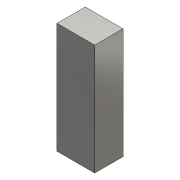
# Autodesk Inventor part: BLANK-BC-10008
Saved by Autodesk Inventor 2016 (Build 200138000, 138)
## iProperties
Created: 2015-12-02
Part Number: BLANK-BC-10008
Material: Aço Carbono
Document SubType Name: Modeling
Designer: reinaldo.basilio
Density: 7.87 g/cm^3
Appearance: Semi-Polished
Mass: 9632.88 g
Surface Area: 798 cm^2
Volume: 1224 cm^3
Project: DIPOLO BC-3T- SIRIUS
Cost Center: 1504002005
Description: Peça frontal inferior para fechar circuito  magnético.
Author: reinaldo.basilio
Title: DIPOLO BC-3T- SIRIUS
Subject: BLANK-BC-10008
Autodesk Inventor part; units mm, degrees
ref_plane "YZ Plane" through (0, 0, 0) normal (1, 0, 0) x (0, 1, 0)
ref_plane "XZ Plane" through (0, 0, 0) normal (0, 1, 0) x (-1, 0, 0)
ref_plane "XY Plane" through (0, 0, 0) normal (0, 0, 1) x (1, 0, 0)
sketch "Sketch1" plane through (0, 0, 0) normal (0, 1, 0) x (-1, 0, 0)
  line L0 (40, 117.5) -> (-40, 117.5)
  line L1 (-40, 117.5) -> (-40, -117.5)
  line L2 (-40, -117.5) -> (40, -117.5)
  line L3 (40, -117.5) -> (40, 117.5)
  point P0 (0, 0)
  point P1 (40, 0)
  point P2 (0, -117.5)
  dimension "d0" = 235
  dimension "d1" = 80
  constraints: 8 end point, 2 midpoint, 2 parallel, 1 horizontal, 1 horizontal alignment, 1 perpendicular, 1 vertical alignment
  measures "d0" distance of L2.end L0.start
  measures "d1" distance of L0.start L0.end
extrude "Extrusion1" add sketch "Sketch1" along normal blind 60
body "Solid1"
